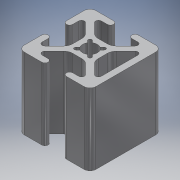
# Autodesk Inventor part: 1003-S
Saved by Autodesk Inventor 2017 SP1 (Build 210196100, 196)
## iProperties
Created: 2016-09-13
Part Number: 1003-S
Material: 6105-T5
Description: 40 S SHORT SINGLE UNIBEARING ASSEMBLY ON 40-4040 X 75mm
Document SubType Name: Modeling
Designer: BRALEF
Density: 1 g/cm^3
Appearance: CLEAR ANODIZED
MATERIAL: 6061-T6
PART PRICE: 44.65
Author: BRALEF
Autodesk Inventor part; units mm, degrees
ref_plane "YZ Plane" through (0, 0, 0) normal (1, 0, 0) x (0, 1, 0)
ref_plane "XZ Plane" through (0, 0, 0) normal (0, 1, 0) x (-1, 0, 0)
ref_plane "XY Plane" through (0, 0, 0) normal (0, 0, 1) x (1, 0, 0)
sketch "Sketch1" plane through (0, 0, 0) normal (0, 1, 0) x (-1, 0, 0)
  arc A0 (2.8605, 1.9692) -> (1.9692, 2.8605) centre (2.4696, 2.4696) ccw
  line L0 (1.3405, 2.2319) -> (1.9692, 2.8605)
  arc A1 (1.3405, 2.2319) -> (-1.3405, 2.2319) centre (0, 0) ccw
  line L1 (-1.9692, 2.8605) -> (-1.3405, 2.2319)
  arc A2 (-1.9692, 2.8605) -> (-2.8605, 1.9692) centre (-2.4696, 2.4696) ccw
  line L2 (-2.2319, 1.3405) -> (-2.8605, 1.9692)
  arc A3 (-2.2319, 1.3405) -> (-2.2319, -1.3405) centre (0, 0) ccw
  line L3 (-2.8605, -1.9692) -> (-2.2319, -1.3405)
  arc A4 (-2.8605, -1.9692) -> (-1.9692, -2.8605) centre (-2.4696, -2.4696) ccw
  line L4 (-1.3405, -2.2319) -> (-1.9692, -2.8605)
  arc A5 (-1.3405, -2.2319) -> (1.3405, -2.2319) centre (0, 0) ccw
  line L5 (1.9692, -2.8605) -> (1.3405, -2.2319)
  arc A6 (1.9692, -2.8605) -> (2.8605, -1.9692) centre (2.4696, -2.4696) ccw
  line L6 (2.2319, -1.3405) -> (2.8605, -1.9692)
  arc A7 (2.2319, -1.3405) -> (2.2319, 1.3405) centre (0, 0) ccw
  line L7 (2.8605, 1.9692) -> (2.2319, 1.3405)
  arc A8 (-4.5172, 1.6401) -> (-5.4471, 3.8852) centre (-7.6922, 1.6401) ccw
  line L8 (-8.7558, 7.1939) -> (-5.4471, 3.8852)
  arc A9 (-8.7558, 7.1939) -> (-10.4905, 6.4753) centre (-9.4743, 6.4753) ccw
  line L9 (-10.4905, -6.4748) -> (-10.4905, 6.4753)
  arc A10 (-10.4905, -6.4748) -> (-8.7558, -7.1933) centre (-9.4743, -6.4748) ccw
  line L10 (-5.4471, -3.8846) -> (-8.7558, -7.1933)
  arc A11 (-5.4471, -3.8846) -> (-4.5172, -1.6396) centre (-7.6922, -1.6396) ccw
  line L11 (-4.5172, 1.6401) -> (-4.5172, -1.6396)
  arc A12 (1.6396, 4.5172) -> (3.8846, 5.4471) centre (1.6396, 7.6922) ccw
  line L12 (3.8846, 5.4471) -> (7.1933, 8.7558)
  arc A13 (7.1933, 8.7558) -> (6.4748, 10.4905) centre (6.4748, 9.4743) ccw
  line L13 (6.4748, 10.4905) -> (4.356, 10.4905)
  arc A14 (4.356, 12.7003) -> (4.356, 10.4905) centre (4.356, 11.5954) ccw
  line L14 (4.356, 12.7003) -> (10.5919, 12.7003)
  arc A15 (12.7001, 10.5921) -> (10.5919, 12.7003) centre (10.5919, 10.5921) ccw
  line L15 (12.7001, 10.5921) -> (12.7001, 4.3562)
  arc A16 (10.4903, 4.3562) -> (12.7001, 4.3562) centre (11.5952, 4.3562) ccw
  line L16 (10.4903, 4.3562) -> (10.4903, 6.475)
  arc A17 (10.4903, 6.475) -> (8.7555, 7.1936) centre (9.4741, 6.475) ccw
  line L17 (8.7555, 7.1936) -> (5.4468, 3.8849)
  arc A18 (5.4468, 3.8849) -> (4.5169, 1.6399) centre (7.6919, 1.6399) ccw
  line L18 (4.5169, 1.6399) -> (4.5169, -1.6396)
  arc A19 (4.5169, -1.6396) -> (5.4468, -3.8846) centre (7.6919, -1.6396) ccw
  line L19 (5.4468, -3.8846) -> (8.7555, -7.1933)
  arc A20 (8.7555, -7.1933) -> (10.4903, -6.4748) centre (9.4741, -6.4748) ccw
  line L20 (10.4903, -6.4748) -> (10.4903, -4.356)
  arc A21 (12.7001, -4.356) -> (10.4903, -4.356) centre (11.5952, -4.356) ccw
  line L21 (12.7001, -4.356) -> (12.7001, -10.5919)
  arc A22 (10.5919, -12.7001) -> (12.7001, -10.5919) centre (10.5919, -10.5919) ccw
  line L22 (10.5919, -12.7001) -> (4.356, -12.7001)
  arc A23 (4.356, -10.4903) -> (4.356, -12.7001) centre (4.356, -11.5952) ccw
  line L23 (4.356, -10.4903) -> (6.475, -10.4903)
  arc A24 (6.475, -10.4903) -> (7.1936, -8.7555) centre (6.475, -9.4741) ccw
  line L24 (7.1936, -8.7555) -> (3.8846, -5.4465)
  arc A25 (3.8846, -5.4465) -> (1.6396, -4.5166) centre (1.6396, -7.6916) ccw
  line L25 (1.6396, -4.5166) -> (-1.6396, -4.5166)
  arc A26 (-1.6396, -4.5166) -> (-3.8846, -5.4465) centre (-1.6396, -7.6916) ccw
  line L26 (-3.8846, -5.4465) -> (-7.1936, -8.7555)
  arc A27 (-7.1936, -8.7555) -> (-6.475, -10.4903) centre (-6.475, -9.4741) ccw
  line L27 (-6.475, -10.4903) -> (-4.3562, -10.4903)
  arc A28 (-4.3562, -12.7001) -> (-4.3562, -10.4903) centre (-4.3562, -11.5952) ccw
  line L28 (-4.3562, -12.7001) -> (-10.5919, -12.7001)
  arc A29 (-12.7001, -10.5919) -> (-10.5919, -12.7001) centre (-10.5919, -10.5919) ccw
  line L29 (-12.7001, -10.5919) -> (-12.7001, 10.5921)
  arc A30 (-10.5919, 12.7003) -> (-12.7001, 10.5921) centre (-10.5919, 10.5921) ccw
  line L30 (-10.5919, 12.7003) -> (-4.3562, 12.7003)
  arc A31 (-4.3562, 10.4905) -> (-4.3562, 12.7003) centre (-4.3562, 11.5954) ccw
  line L31 (-4.3562, 10.4905) -> (-6.475, 10.4905)
  arc A32 (-6.475, 10.4905) -> (-7.1936, 8.7558) centre (-6.475, 9.4743) ccw
  line L32 (-7.1936, 8.7558) -> (-3.8849, 5.4471)
  arc A33 (-3.8849, 5.4471) -> (-1.6399, 4.5172) centre (-1.6399, 7.6922) ccw
  line L33 (-1.6399, 4.5172) -> (1.6396, 4.5172)
  point P0 (0, 0)
  dimension "d36" = 8.1835
  dimension "d81" = 1.0162
  dimension "d82" = 3.175
  dimension "d95" = 8.1832
  dimension "d96" = 17.2172
  dimension "d97" = 23.1906
  dimension "d98" = 25.4002
  dimension "d100" = 8.1832
  dimension "d101" = 2.2092
  dimension "d104" = 2.2091
  dimension "d131" = 1.1049
  dimension "d132" = 2.1082
  dimension "d133" = 0.635
  dimension "d134" = 2.6035
  dimension "d135" = 2.6035
  dimension "d136" = 2.6035
  dimension "d137" = 2.6035
  dimension "d138" = 45
  dimension "d139" = 45
  dimension "d140" = 45
  dimension "d141" = 45
  dimension "d142" = 45
  dimension "d143" = 25.4004
  dimension "d144" = 0.4742
  dimension "d145" = 1.7347
  dimension "d146" = 0.4744
  dimension "d147" = 1.7349
  dimension "d148" = 12.7001
  dimension "d149" = 12.7003
  dimension "d150" = 1.1046
  dimension "d151" = 1.1048
  dimension "d152" = 0.6303
  dimension "d153" = 0.6303
  dimension "d154" = 0.6303
  dimension "d155" = 0.6303
  dimension "d156" = 8.3441
  dimension "d157" = 17.0563
  dimension "d158" = 8.3441
  dimension "d159" = 8.3441
  dimension "d160" = 9.8396
  dimension "d161" = 9.8396
  dimension "d162" = 10.2305
  dimension "d163" = 10.2305
  dimension "d164" = 10.4682
  dimension "d165" = 10.4682
  dimension "d166" = 14.6692
  dimension "d167" = 14.6692
  dimension "d168" = 15.1696
  dimension "d169" = 15.1696
  dimension "d170" = 17.0563
  dimension "d171" = 17.0563
  constraints: 72 tangent, 68 end point, 68 point on circle, 34 centre point, 22 equal radius, 16 parallel, 1 horizontal, 1 perpendicular, 1 vertical
  measures "d36" distance between parallel lines of L22 L25
  measures "d81" radius of A17
  measures "d82" radius of A18
  measures "d95" distance between parallel lines of L21 L18
  measures "d96" distance between parallel lines of L21 L11
  measures "d97" distance between parallel lines of L21 L9
  measures "d98" distance between parallel lines of L21 L29
  measures "d100" distance between parallel lines of L14 L33
  measures "d101" distance between parallel lines of L17 L12
  measures "d104" distance between parallel lines of L19 L24
  measures "d131" radius of A16
  measures "d132" radius of A15
  measures "d133" radius of A0
  measures "d134" radius of A7
  measures "d135" radius of A1
  measures "d136" radius of A5
  measures "d137" radius of A3
  measures "d138" angle of L17 L21
  measures "d139" angle of L7 L21
  measures "d140" angle of L15 L6
  measures "d141" angle of L15 L0
  measures "d142" angle of L5 L21
  measures "d143" distance between parallel lines of L22 L14
  measures "d144" distance between parallel lines of L4 L17
  measures "d145" distance between parallel lines of L3 L17
  measures "d146" distance between parallel lines of L1 L19
  measures "d147" distance between parallel lines of L2 L19
  measures "d148" distance from line of point (0, 0) L21
  measures "d149" distance from line of point (0, 0) L14
  measures "d150" distance from line of point (0, 0) L19
  measures "d151" distance from line of point (0, 0) L12
  measures "d152" distance from line of point (0, 0) L7
  measures "d153" distance from line of point (0, 0) L6
  measures "d154" distance from line of point (0, 0) L0
  measures "d155" distance from line of point (0, 0) L5
  measures "d156" distance from line of L15.end L14
  measures "d157" distance from line of L21.start L14
  measures "d158" distance from line of L14.start L21
  measures "d159" distance from line of L23.start L21
  measures "d160" distance from line of L7.start L21
  measures "d161" distance from line of L6.end L21
  measures "d162" distance from line of A0.centre L21
  measures "d163" distance from line of A6.centre L21
  measures "d164" distance from line of L7.end L21
  measures "d165" distance from line of L6.start L21
  measures "d166" distance from line of L1.start L21
  measures "d167" distance from line of L4.end L21
  measures "d168" distance from line of A2.centre L21
  measures "d169" distance from line of A4.centre L21
  measures "d170" distance from line of L30.end L21
  measures "d171" distance from line of L27.end L21
extrude "Extrusion1" add sketch "Sketch1" along normal mid plane 25.4
body "Solid1"
